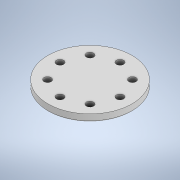
# Autodesk Inventor part: kiść
Saved by Autodesk Inventor 2021 (Build 250183000, 183)
## iProperties
Created: 2021-11-09
Part Number: kiść
Material: Generic
Document SubType Name: Modeling
Designer: Łukasz
Density: 1 g/cm^3
Appearance: Default
Author: Łukasz
Autodesk Inventor part; units mm, degrees
ref_plane "YZ Plane" through (0, 0, 0) normal (1, 0, 0) x (0, 1, 0)
ref_plane "XZ Plane" through (0, 0, 0) normal (0, 1, 0) x (-1, 0, 0)
ref_plane "XY Plane" through (0, 0, 0) normal (0, 0, 1) x (1, 0, 0)
sketch "Sketch1" plane through (0, 0, 0) normal (0, 0, 1) x (1, 0, 0)
  line L0 (0, 0) -> (-14, 0)
  line L1 (-35, 0) -> (-35, 5)
  line L2 (-35, 5) -> (0, 5)
  line L3 (35, 5) -> (35, 0)
  line L4 (0, -10) -> (-14, -10)
  line L5 (-14, -10) -> (-14, -5)
  line L6 (-14, -5) -> (0, -5)
  line L7 (14, -5) -> (14, -10)
  spline S0 degree 3 poles (-14, -5) (-15.7698, -2.5106) (-33.5733, -3.9868) (-35, 0) knots 0 0 0 0 1 1 1 1
  line L8 (0, -10) -> (0, 5)
  point P0 (0, 0)
  point P1 (-18.2816, -3.6679)
  point P2 (-30.5642, -2.2908)
  dimension "d0" = 70
  dimension "d1" = 5
  dimension "d2" = 35
  dimension "d3" = 28
  dimension "d4" = 5
  dimension "d5" = 14
  dimension "d6" = 5
  constraints: 18 end point, 4 parallel, 3 point on line, 2 horizontal, 2 perpendicular, 4 other
  measures "d0" distance of L1.end L3.start
  measures "d1" distance of L1.start L1.end
  measures "d2" distance from line of point (0, 0) L3
  measures "d3" distance of L5.end L7.start
  measures "d4" distance of L4.end L5.end
  measures "d5" distance from line of point (0, 0) L7
  measures "d6" distance between parallel lines of L0 L6
revolve "Revolution1" add sketch "Sketch1" angle 360 about axis through (0, -10, 0) along (0, 1, 0)
fillet "Fillet1" radius 5 1 edges at (14, -5, 0)
sketch "Sketch2" plane through (0, -10, 0) normal (0, -1, 0) x (1, 0, 0)
  circle A0 centre (0, 0) radius 10.5
  dimension "d9" = 21
  constraints: 1 centre point, 1 coincident
  measures "d9" diameter of A0
extrude "Extrusion1" cut sketch "Sketch2" against normal blind 2.5
sketch "Sketch3" plane through (0, 5, 0) normal (0, 1, 0) x (1, 0, 0)
  circle A0 centre (0, -25) radius 3
  circle A1 centre (17.6777, -17.6777) radius 3
  circle A2 centre (25, 0) radius 3
  circle A3 centre (17.6777, 17.6777) radius 3
  circle A4 centre (0, 25) radius 3
  circle A5 centre (-17.6777, 17.6777) radius 3
  circle A6 centre (-25, 0) radius 3
  circle A7 centre (-17.6777, -17.6777) radius 3
  point P0 (0, 0)
  point P1 (0, 0)
  point P2 (0, 0)
  point P3 (0, 0)
  point P4 (0, 0)
  point P5 (0, 0)
  point P6 (0, 0)
  point P7 (0, 0)
  dimension "d12" = 6
  dimension "d13" = 25
  dimension "d16" = 360
  constraints: 8 centre point, 2 coincident, 23 other
  measures "d12" diameter of A0
  measures "d13" distance of point (0, 0) A0.centre
extrude "Extrusion2" cut sketch "Sketch3" against normal blind 10
body "Solid1"
